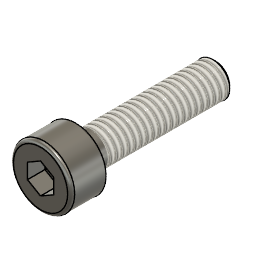
_8KEYWE6RKB4RY3AVARTBXGBUTen-US11.58c39408-2f88-4fb6-8834-311d7a520ea7 (Autodesk Fusion 360 design; units mm, degrees)
description: Hexagon Socket Head Cap Screw STN EN ISO 4762 - M4 x 16
part number: STN EN ISO 4762 - M4 x 16 Steel 4.6 Plain
Autodesk Fusion 360 part; units mm, degrees
sketch "Sketch1" plane through (0, 0, 0) normal (0, 1, 0) x (1, 0, 0)
  line L0 (-2, 0) -> (-2, 16)
  line L1 (-2, 16) -> (0, 16)
  line L2 (0, 16) -> (0, -4)
  line L3 (-2, 0) -> (-3.5, 0)
  line L4 (-3.5, 0) -> (-3.5, -4)
  line L5 (-3.5, -4) -> (0, -4)
  dimension "d9" = 4
  dimension "d106" = 4
  dimension "d107" = 16
  dimension "d116" = 7
  constraint perpendicular L0 L1
  constraint collinear origin L1.end L2.end
  constraint perpendicular L0 L3
  constraint coincident origin L3
  constraint vertical L2
  constraint coincident L2 L5.end
  constraint perpendicular L2 L5
  measures "d106" distance of L3 L5
  measures "d107" distance of origin L1
revolve "Revolve1" add sketch "Sketch1" angle 360 about axis through (0, 0, -16) along (0, 0, 1)
ref_plane "WorkPlane1" through (0, 0, 4) normal (0, 0, 1) x (1, 0, 0)
sketch "Sketch6" plane through (0, 0, 4) normal (0, 0, 1) x (1, 0, 0)
  line L0 (-1.5, 0.866) -> (-1.5, -0.866)
  line L1 (-1.5, -0.866) -> (0, -1.7321)
  line L2 (0, -1.7321) -> (1.5, -0.866)
  line L3 (1.5, -0.866) -> (1.5, 0.866)
  line L4 (1.5, 0.866) -> (0, 1.7321)
  line L5 (0, 1.7321) -> (-1.5, 0.866)
  dimension "d117" = 3
  constraint vertical L0
  measures "d117" distance of L0 L3
extrude "Extrude1" cut sketch "Sketch6" against normal blind 2
extrude "Extrude2" cut 1 faces at (-0.5, -0.2887, 2) along direction (0, 0, -1) blind 2 draft -85
fillet "Fillet4" radius 0.4 1 edges at (-3.2631, 1.2657, 4)
thread "Thread3" "ISO Metric profile 4.0 M4x0.7 M4x0.7 6g" major diameter 3.908 minor diameter 3.111 pitch 0.7 angle 60 resizes the face on face at (-1.9901, 0.1991, -10.6667) from (0, 0, -1.75) to (0, 0, -16)
sketch "Sketch7" plane through (0, 0, 0) normal (0, 1, 0) x (1, 0, 0)
  line L0 (-2.04, 16) -> (-2.04, 15.6)
  line L1 (-2.04, 15.6) -> (-1.64, 16)
  line L2 (0, 16) -> (0, -4)
  line L3 (-2.04, 16) -> (0, 16)
  dimension "d101" = 45
  dimension "d112" = 0.4
  dimension "d113" = 2.04
  constraint coincident L2.start L3.end
  constraint perpendicular L2 L3
  constraint coincident L1.end L3
  constraint perpendicular L0 L3
  measures "d101" angle of L0 L1
  measures "d112" distance of L0.end L3
  measures "d113" distance of L0 L2.start
revolve "Revolve3" cut sketch "Sketch7" angle 360 about axis through (0, 0, 1.75) along (0, 0, 1)
equation "d9 = adsk_nomdia"
equation "adsk_nomlen = 16.00 mm"
equation "adsk_headh = 4.00 mm"
equation "adsk_headdia = 7.00 mm"
equation "adsk_nomdia = 4.00 mm"
equation "adsk_philwidth = 3.00 mm"
equation "d31 = -adsk_phildepth"
equation "adsk_phildepth = 2.00 mm"
equation "d71 = adsk_headh"
equation "d76 = -adsk_phildepth"
equation "adsk_thrlen = 14.25 mm"
equation "d86 = adsk_nomdia * 0.1"
equation "adsk_startang = 45.00 deg"
equation "d101 = adsk_startang"
equation "adsk_pitch1 = 0.70 mm"
equation "adsk_startlen = 0.40 mm"
equation "d106 = adsk_headh"
equation "d107 = adsk_nomlen"
equation "d112 = adsk_startlen"
equation "d113 = adsk_nomdia * 0.51"
equation "d115 = min(adsk_thrlen; adsk_nomlen - 0.001 mm)"
equation "d116 = adsk_headdia"
equation "d117 = adsk_philwidth"
